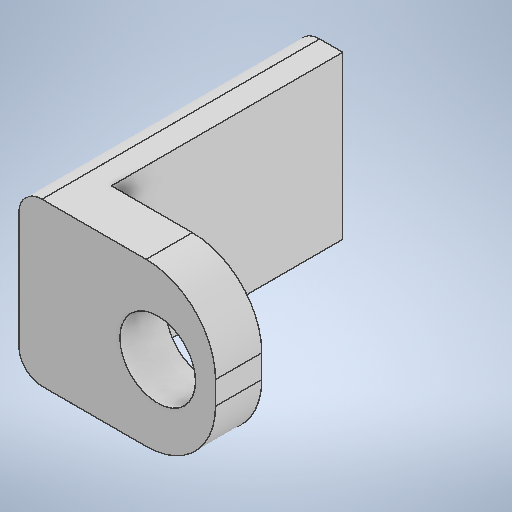
# Autodesk Inventor part: guide_link
Saved by Autodesk Inventor 2025 (Build 290162000, 162)
## iProperties
Created: 2025-09-16
Part Number: guide_link
Material: 一般
Document SubType Name: Modeling
Designer: sooo1
Density: 1 g/cm^3
Appearance: 既定
Author: sooo1
Autodesk Inventor part; units mm, degrees
ref_plane "YZ Plane" through (0, 0, 0) normal (1, 0, 0) x (0, 1, 0)
ref_plane "XZ Plane" through (0, 0, 0) normal (0, 1, 0) x (-1, 0, 0)
ref_plane "XY Plane" through (0, 0, 0) normal (0, 0, 1) x (1, 0, 0)
sketch "スケッチ1" plane through (0, 0, 0) normal (0, 0, 1) x (1, 0, 0)
  circle A0 centre (0, 0) radius 1.635
  line L0 (-6, -3.5) -> (2.5, -3.5)
  line L1 (2.5, -3.5) -> (2.5, 3.5)
  line L2 (2.5, 3.5) -> (-6, 3.5)
  line L3 (-6, 3.5) -> (-6, -3.5)
  line L4 (-6, -3.5) -> (2.5, 3.5) construction
  line L5 (2.5, -3.5) -> (-6, 3.5) construction
  line L6 (-6, 0) -> (2.5, 0) construction
  line L7 (-4, 3.5) -> (-4, -3.5)
  point P0 (-1.75, 0)
  dimension "d0" = 3.27
  dimension "d1" = 7
  dimension "d2" = 2.5
  dimension "d3" = 6
  dimension "d6" = 2
  constraints: 16 end point, 4 midpoint, 3 point on line, 2 parallel, 2 perpendicular, 1 centre point, 1 coincident, 1 horizontal
  measures "d0" diameter of A0
  measures "d1" distance of L2.end L0.start
  measures "d2" distance from line of L1 A0.centre
  measures "d3" distance from line of A0.centre L3
  measures "d6" distance between parallel lines of L3 L7
extrude "押し出し1" add sketch "スケッチ1" along normal blind 2
extrude "押し出し2" add sketch "スケッチ1" against normal blind 10 contours L3 L2 L7 L0
fillet "フィレット1" radius 3 2 edges at (2.5, 3.5, 1) (2.5, -3.5, 1)
fillet "フィレット2" radius 1 2 edges at (-6, -3.5, -4) (-6, 3.5, -4)
